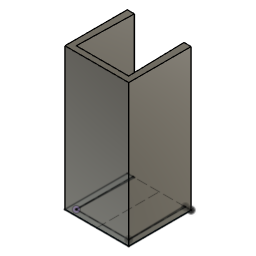
Table Distance Keeper v4 (Autodesk Fusion 360 design; units mm, degrees)
Autodesk Fusion 360 part; units mm, degrees
sketch "Schizzo1" plane through (0, 0, 0) normal (0, 0, 1) x (1, 0, 0)
  line L0 (0, 0) -> (18.5, 0) construction
  line L1 (18.5, 0) -> (18.5, 20) construction
  line L2 (18.5, 20) -> (0, 20) construction
  line L3 (0, 20) -> (0, 0) construction
  line L4 (20.5, -2) -> (20.5, 20)
  line L5 (-2, 20) -> (-2, -2)
  line L6 (-2, -2) -> (20.5, -2)
  line L7 (-2, 20) -> (0, 20)
  line L8 (0, 20) -> (0, 0)
  line L9 (0, 0) -> (18.5, 0)
  line L10 (18.5, 0) -> (18.5, 20)
  line L11 (18.5, 20) -> (20.5, 20)
  line L12 (0, 20) -> (0.5, 20)
  line L13 (0, 0) -> (0.5, 20)
  line L14 (9.25, -2) -> (9.25, 20) construction
  line L15 (18.5, 0) -> (18, 20)
  line L16 (18.5, 20) -> (18, 20)
  point P0 (20.5, 20)
  dimension "d1" = 18.5
  dimension "d2" = 20
  dimension "d6" = 0.5
  constraint horizontal L0
  constraint vertical L1
  constraint horizontal L2
  constraint vertical L3
  constraint coincident L0.start L3.end
  constraint perpendicular L3 L7
  constraint perpendicular L4 L11
  constraint perpendicular L8 L12
  constraint midpoint L6 L14.start
  constraint midpoint L2 L14.end
  constraint symmetric L0.start L14 L0.end
  constraint symmetric L2.end L14 L1.end
  constraint symmetric L5.start L14 P0
  constraint symmetric L12.end L14 L15.end
  measures "d1" distance of L0.start L0.end
  measures "d2" distance of L0 L2
  measures "d6" distance of L2.end L12.end
extrude "Estrusione1" add sketch "Schizzo1" along normal blind 50
sketch "Schizzo2" plane through (20.5, 0, 0) normal (1, 0, 0) x (0, 1, 0)
  line L0 (-2, 0) -> (20, 0)
  line L1 (20, 0) -> (20, 50)
  line L2 (20, 50) -> (-2, 50)
  line L3 (-2, 50) -> (-2, 0)
  line L4 (-2, 25) -> (20, 25) construction
  line L5 (-2, 0) -> (20, 0) construction
  line L6 (-2, 25) -> (20, 25)
  line L7 (20, 25) -> (20, 0)
  line L8 (20, 0) -> (-2, 0)
  line L9 (-2, 0) -> (-2, 25)
  dimension "d7" = 25
  constraint coincident L3 L4.start
  constraint coincident L1 L4.end
  constraint perpendicular L1 L4
  constraint horizontal L6
  constraint vertical L7
  constraint horizontal L8
  constraint vertical L9
  constraint coincident L0.end L1.start
  measures "d7" distance of L4 L5
extrude "Estrusione2" add sketch "Schizzo2" against normal blind 22 contours L0 L1 L3 L6 L7 L8 L9
